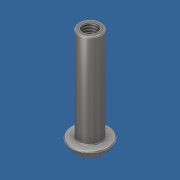
# Autodesk Inventor part: Axel-Female
Saved by Autodesk Inventor 2018 (Build 220112000, 112)
## iProperties
Created: 2018-03-01
Part Number: Axel-Female
Material: Stainless Steel
Document SubType Name: Modeling
Designer: 232963
Density: 8 g/cm^3
Appearance: Semi-Polished
Mass: 12.2274 g
Surface Area: 15.6803 cm^2
Volume: 1.52843 cm^3
Author: 232963
Autodesk Inventor part; units mm, degrees
ref_plane "YZ Plane" through (0, 0, 0) normal (1, 0, 0) x (0, 1, 0)
ref_plane "XZ Plane" through (0, 0, 0) normal (0, 1, 0) x (-1, 0, 0)
ref_plane "XY Plane" through (0, 0, 0) normal (0, 0, 1) x (1, 0, 0)
sketch "Sketch1" plane through (0, 0, 0) normal (0, 0, 1) x (1, 0, 0)
  line L0 (0, 0) -> (0, 38.608)
  line L1 (0, 38.608) -> (3.9116, 38.608)
  line L2 (3.9116, 38.608) -> (3.9116, 5.1562)
  line L3 (3.9116, 5.1562) -> (6.731, 5.1562)
  line L4 (6.731, 5.1562) -> (3.9116, 5.1562)
  line L5 (6.731, 5.1562) -> (3.9116, 5.1562)
  arc A0 (0, 0) -> (6.731, 5.1562) centre (0, 6.9715) ccw
  dimension "d0" = 38.608
  dimension "d1" = 6.731
  dimension "d3" = 3.9116
  dimension "d4" = 33.4518
  constraints: 12 end point, 3 perpendicular, 3 point on circle, 1 centre point, 1 point on line, 1 vertical
  measures "d0" distance of L0.start L0.end
  measures "d1" distance from line of L3.end L0
  measures "d3" distance of L0.end L1.end
  measures "d4" distance of L2.end L1.end
revolve "Revolution1" add sketch "Sketch1" angle 360 about axis through (0, 0, 0) along (0, 1, 0)
fillet "Fillet1" radius 0.3175 1 edges at (-6.731, 5.1562, 0)
sketch "Sketch2" plane through (0, 5.1562, 0) normal (0, 1, 0) x (1, 0, 0)
  point P0 (0, 0)
ref_plane "Work Plane1" through (0, 0.3937, 0) normal (0, 1, 0) x (1, 0, 0)
sketch "Sketch3" plane through (0, 0.3937, 0) normal (0, 1, 0) x (1, 0, 0)
  line L0 (0, 2.8575) -> (2.4747, 1.4287)
  line L1 (2.4747, 1.4287) -> (2.4747, -1.4287)
  line L2 (2.4747, -1.4287) -> (0, -2.8575)
  line L3 (0, -2.8575) -> (-2.4747, -1.4288)
  line L4 (-2.4747, -1.4288) -> (-2.4747, 1.4287)
  line L5 (-2.4747, 1.4287) -> (0, 2.8575)
  point P0 (0, 0)
  point P1 (0, 0)
  dimension "d9" = 5.715
  constraints: 12 end point, 1 coincident, 13 other
  measures "d9" distance of L0.start L2.end
extrude "Extrusion1" cut sketch "Sketch3" along normal blind 4.572 and the other way blind 2.286
fillet "Fillet2" radius 0.3175 1 edges at (-3.9116, 5.1562, 0)
fillet "Fillet3" radius 0.3175 1 edges at (-3.9116, 38.608, 0)
sketch "Sketch4" plane through (0, 38.608, 0) normal (0, 1, 0) x (1, 0, 0)
  circle A0 centre (0, 0) radius 3.5941 projected
  circle A1 centre (0, 0) radius 2.6035
  dimension "d16" = 5.207
  constraints: 1 centre point, 1 coincident
  measures "d16" diameter of A1
extrude "Extrusion2" cut sketch "Sketch4" against normal blind 19.558 contours A1
thread "Thread1" size "1/4-28 UNF" class "2B" standard "ANSI Unified Screw Threads" full length
body "Solid1"
